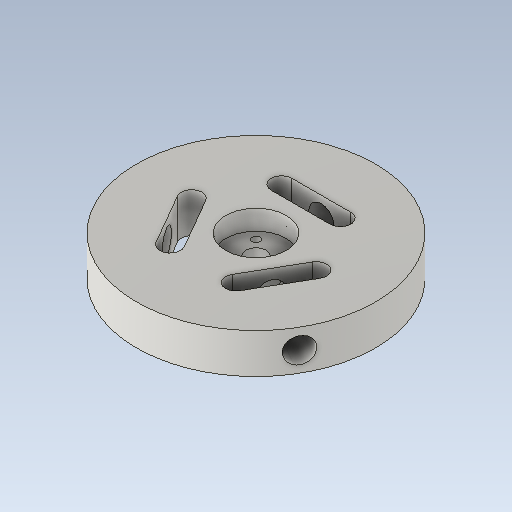
# Autodesk Inventor part: PWTR-0032
Saved by Autodesk Inventor 2021.1 (Build 251245010, 245A)
## iProperties
Part Number: PWTR-0032
Document SubType Name: Modeling
Created: 2003-02-04
Designer: B. BOGAN
Material: Aluminum-6061
Description: Trowel Spider
Density: 2.71 g/cm^3
Appearance: Steel
Mass: 896.99 g
Surface Area: 624.47 cm^2
Volume: 330.993 cm^3
Vendor: Design Specific
Control State: 0
Master: False
Checked Out: False
Shininess: 64.0
Length Units: 11269
Angle Units: 11279
Time Units: 11290
Mass Units: 11284
Length Display Precision: 3
Angle Display Precision: 2
Compacted: True
Density: 0.0
Volumn: 0.0
Area: 0.0
PropertySet Name: Model Information
Title: TROWEL SPIDER
Author: B. BOGAN
Revision Number: B
Autodesk Inventor part; units mm, degrees
ref_plane "XZ Plane" through (0, 0, 0) normal (0, 1, 0) x (-1, 0, 0)
ref_plane "XY Plane" through (0, 0, 0) normal (0, 0, 1) x (1, 0, 0)
sketch "Sketch1" plane through (0, 0, 0) normal (0, 0, 1) x (1, 0, 0)
  circle A0 centre (0, 0) radius 75
  dimension "d114" = 150
  constraints: 1 centre point, 1 coincident
  measures "d114" diameter of A0
extrude "Extrusion1" add sketch "Sketch1" along normal blind 25
ref_plane "HoleTangent" through (75, 0, 0) normal (1, 0, 0) x (0, 1, 0)
sketch "Sketch3" plane through (0, 0, 25) normal (0, 0, 1) x (1, 0, 0)
  point P0 (0, 0)
  point P1 (0, 0)
  constraints: 1 coincident
hole "Hole1" at (0, 0, 25) direction (0, 0, -1) diameter 12.7 end through all
sketch "Sketch6" plane through (0, 0, 25) normal (0, 0, 1) x (1, 0, 0)
  circle A0 centre (0, 0) radius 6.35 projected
  circle A1 centre (0, 0) radius 19.05
  dimension "d46" = 38.1
  constraints: 1 centre point, 1 coincident
  measures "d46" diameter of A1
extrude "Extrusion4" cut sketch "Sketch6" against normal blind 12.5
sketch "Sketch7" plane through (0, 0, 0) normal (0, 0, -1) x (-1, 0, 0)
  circle A0 centre (0, 0) radius 6.35 projected
  circle A1 centre (0, 0) radius 12.7 construction
  line L0 (0, 0) -> (8.9803, 8.9803) construction
  line L1 (0, 0) -> (11.1003, 0) construction
  dimension "d49" = 25.4
  dimension "d50" = 45
  constraints: 4 end point, 2 coincident, 3 other
  measures "d50" angle of L0 L1
hole "Hole3" at (-8.9803, 8.9803, 0) direction (0, 0, 1) diameter 5.08 end through all
pattern_circular "Circular Pattern3" count 4 over 360 about axis through (0, 0, -188.6001) along (0, 0, 1) of "Hole3"
sketch "Sketch5" plane through (75, 12.7, 25.4) normal (1, 0, 0) x (0, 0, -1)
  line L0 (30.48, -12.7) -> (-5.08, -12.7) projected
  point P0 (12.9, -12.7)
  point P1 (25.4, -12.7)
  dimension "d116" = 12.5
  constraints: 1 point on line
  measures "d116" distance of point (25.4, -12.7) point (12.9, -12.7)
hole "Hole2" at (75, 0, 12.5) direction (-1, 0, 0) diameter 12.7 depth 55.5625 counterbore diameter 15.875 counterbore depth 34.925
sketch "Sketch4" plane through (0, 0, 25) normal (0, 0, 1) x (1, 0, 0)
  line L0 (41, 18.5) -> (41, -18.5)
  line L1 (28, -18.5) -> (28, 18.5)
  arc A0 (41, 18.5) -> (28, 18.5) centre (34.5, 18.5) ccw
  arc A1 (28, -18.5) -> (41, -18.5) centre (34.5, -18.5) ccw
  circle A2 centre (0, 0) radius 19.05 projected
  point P0 (28, 0)
  dimension "d22" = 50
  dimension "d24" = 6.5
  dimension "d62" = 34.5
  constraints: 4 end point, 4 point on circle, 4 tangent, 2 centre point, 1 horizontal alignment, 1 midpoint, 1 parallel, 1 vertical
  measures "d24" radius of A0
  measures "d62" horizontal distance of A1.centre A2.centre
extrude "Extrusion3" cut sketch "Sketch4" against normal through all contours L0 A1 L1 A0
pattern_circular "Circular Pattern2" count 3 over 360 about axis through (0, 0, -188.6001) along (0, 0, 1) of "Hole2", "Extrusion3"
sketch "Sketch8" plane through (0, 0, 25) normal (0, 0, 1) x (1, 0, 0)
  line L0 (-10.3502, -47.1424) -> (10.8733, -47.1424) construction
  line L1 (10.8733, -47.1424) -> (10.8733, -60.9041) construction
  line L2 (10.8733, -60.9041) -> (-10.3502, -60.9041) construction
  line L3 (-10.3502, -60.9041) -> (-10.3502, -47.1424) construction
  point P0 (0, 0)
  constraints: 2 other
hole "Hole4" at (75, 0, 12.5) direction (-1, 0, 0) diameter 22.5 depth 2
equation "\"d116\" = 0.5 * d2"
equation "\"d115\" = 0.5 * d114"
equation "\"d2\" = 25"
body "Solid1"
